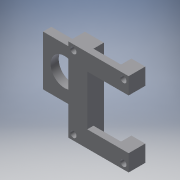
# Autodesk Inventor part: Bat_fixture
Saved by Autodesk Inventor 2019.3 (Build 233278000, 278)
## iProperties
Created: 2020-09-10
Part Number: Bat_fixture
Material: Generisch
Document SubType Name: Modeling
Designer: Nicolas Frick
Density: 1 g/cm^3
Appearance: Vorgabe
Author: Nicolas Frick
Autodesk Inventor part; units mm, degrees
ref_plane "YZ Plane" through (0, 0, 0) normal (1, 0, 0) x (0, 1, 0)
ref_plane "XZ Plane" through (0, 0, 0) normal (0, 1, 0) x (-1, 0, 0)
ref_plane "XY Plane" through (0, 0, 0) normal (0, 0, 1) x (1, 0, 0)
sketch "Skizze1" plane through (0, 0, 0) normal (0, 0, 1) x (1, 0, 0)
  line L0 (7.35, 100) -> (-7.35, 100) construction
  line L1 (-7.35, 0) -> (-7.35, 100) construction
  line L2 (7.35, 0) -> (-7.35, 0) construction
  line L3 (7.35, 0) -> (7.35, 100) construction
  circle A0 centre (-1.15, 77.5) radius 5.5 construction
  circle A1 centre (-1.15, 22.5) radius 5.5 construction
  circle A2 centre (-1.15, 93.5) radius 3.3 construction
  circle A3 centre (-1.15, 6.5) radius 3.3 construction
  line L4 (65.05, 100) -> (50.35, 100) construction
  line L5 (50.35, 0) -> (50.35, 100) construction
  line L6 (65.05, 0) -> (50.35, 0) construction
  line L7 (65.05, 0) -> (65.05, 100) construction
  circle A4 centre (58.85, 77.5) radius 5.5 construction
  circle A5 centre (58.85, 22.5) radius 5.5 construction
  circle A6 centre (58.85, 93.5) radius 3.3 construction
  circle A7 centre (58.85, 6.5) radius 3.3 construction
  line L8 (15.4049, 37.5868) -> (15.4049, 77.5868) construction
  line L9 (42.4049, 37.5868) -> (42.4049, 77.5868) construction
  line L10 (-7.35, 100) -> (65.05, 100)
  line L11 (65.05, 100) -> (65.05, 80)
  line L12 (65.05, 80) -> (-7.35, 80)
  line L13 (-7.35, 80) -> (-7.35, 100)
  line L14 (65.05, 0) -> (-7.35, 0)
  line L15 (-7.35, 0) -> (-7.35, 20)
  line L16 (-7.35, 20) -> (65.05, 20)
  line L17 (65.05, 20) -> (65.05, 0)
  circle A8 centre (-26.825, 50.9692) radius 16.4871 construction
  line L18 (15.4049, 80) -> (-52.5951, 80)
  line L19 (-52.5951, 80) -> (-52.5951, 20)
  line L20 (-52.5951, 20) -> (15.4049, 20)
  line L21 (15.4049, 20) -> (15.4049, 80)
  circle A9 centre (-26.825, 50.9692) radius 16.7
  point P0 (0, 0)
  point P1 (16.9249, 55.5859)
  dimension "d3" = 33.4
  constraints: 24 end point, 6 parallel, 4 point on line, 3 horizontal, 3 perpendicular, 1 centre point, 1 coincident, 1 other
  measures "d3" diameter of A9
extrude "Extrusion1" add sketch "Skizze1" along normal blind 20
sketch "Skizze2" plane through (0, 0, 20) normal (0, 0, 1) x (1, 0, 0)
  circle A0 centre (-1.15, 93.5) radius 2.5 projected
  circle A1 centre (58.85, 93.5) radius 2.5 projected
  circle A2 centre (-1.15, 6.5) radius 2.5 projected
  circle A3 centre (58.85, 6.5) radius 2.5 projected
  point P0 (0, 0)
hole "Bohrung1" at (-1.15, 93.5, 20) at (58.85, 93.5, 20) at (58.85, 6.5, 20) at (-1.15, 6.5, 20) direction (0, 0, -1) diameter 4.3 end through all counterbore diameter 7.3 counterbore depth 7.5
sketch "Skizze3" plane through (-7.35, 0, 0) normal (0, -1, 0) x (1, 0, 0)
  line L0 (46.2, -6) -> (72.4, -6) construction
  line L1 (72.7, -7.2) -> (72.7, -21.5) construction
  line L2 (46.7, -7.2) -> (46.7, -16.5) construction
  line L3 (25.7, -7.2) -> (25.7, -16.5) construction
  line L4 (-0.3, -7.2) -> (-0.3, -21.5) construction
  line L5 (116.8014, -58) -> (115.3014, -58) projected
  line L6 (72.4, 0) -> (57.7, 0) construction
  line L7 (14.7, 0) -> (0, 0) construction
  line L8 (72.4, 0) -> (0, 0) construction
  line L9 (2.55, 20) -> (9.85, 20) construction
  line L10 (62.55, 20) -> (69.85, 20) construction
  line L11 (49.7549, 2.5) -> (49.7549, 8.5) construction
  line L12 (48.2349, 2.5) -> (49.5076, 2.5) construction
  line L13 (72.4, 0) -> (0, 0) construction
  line L14 (72.4, 0) -> (72.4, 20) construction
  line L15 (0, 20) -> (72.4, 20) construction
  line L16 (0, 0) -> (0, 20) construction
  line L17 (22.7549, 8.6) -> (22.7549, 2.6) construction
  line L18 (23.1949, 8.9) -> (51.1949, 8.9) construction
  line L19 (51.1949, 1.6) -> (23.1949, 1.6) construction
  line L20 (55.7549, 12.5) -> (43.7549, 12.5)
  line L21 (0, 0) -> (72.4, 0) construction
  line L22 (43.7549, -12.5) -> (55.7549, 12.5) construction
  line L23 (55.7549, -12.5) -> (43.7549, 12.5) construction
  line L24 (43.7549, 0) -> (55.7549, 0)
  line L25 (55.7549, 0) -> (55.7549, 12.5)
  line L26 (22.7549, 0) -> (43.7549, 0)
  line L27 (43.7549, 12.5) -> (22.7549, 12.5)
  line L28 (22.7549, 12.5) -> (22.7549, 0)
  line L29 (22.7549, 12.5) -> (55.7549, 12.5)
  line L30 (55.7549, 12.5) -> (55.7549, 0)
  line L31 (55.7549, 0) -> (22.7549, 0)
  line L32 (22.7549, 0) -> (22.7549, 12.5)
  point P0 (7.35, 0)
  point P1 (49.7549, 0)
  constraints: 24 end point, 3 parallel, 2 horizontal, 2 midpoint, 1 perpendicular, 5 other
extrude "Extrusion2" cut sketch "Skizze3" against normal through all
sketch "Skizze4" plane through (0, 0, 20) normal (0, 0, 1) x (1, 0, 0)
  circle A0 centre (58.85, 6.5) radius 3.65 construction
  circle A1 centre (-1.15, 93.5) radius 3.65 construction
  circle A2 centre (58.85, 93.5) radius 3.65 construction
  circle A3 centre (-1.15, 6.5) radius 3.65 construction
  circle A4 centre (-26.825, 50.9692) radius 16.7 construction
  line L0 (65.05, 100) -> (-7.35, 100) construction
  line L1 (-7.35, 100) -> (-7.35, 80) construction
  line L2 (-7.35, 80) -> (-52.5951, 80) construction
  line L3 (-52.5951, 80) -> (-52.5951, 20) construction
  line L4 (-52.5951, 20) -> (-7.35, 20) construction
  line L5 (-7.35, 20) -> (-7.35, 0) construction
  line L6 (-7.35, 0) -> (65.05, 0) construction
  line L7 (65.05, 0) -> (65.05, 20) construction
  line L8 (65.05, 20) -> (15.4049, 20) construction
  line L9 (15.4049, 20) -> (15.4049, 80) construction
  line L10 (15.4049, 80) -> (65.05, 80) construction
  line L11 (65.05, 80) -> (65.05, 100) construction
  line L12 (-52.5951, 80) -> (-7.35, 80)
  line L13 (-7.35, 80) -> (-7.35, 20)
  line L14 (-7.35, 20) -> (-52.5951, 20)
  line L15 (-52.5951, 20) -> (-52.5951, 80)
  point P0 (0, 0)
  constraints: 8 end point, 2 parallel, 1 horizontal, 1 perpendicular
extrude "Extrusion3" cut sketch "Skizze4" against normal blind 15
sketch "Skizze5" plane through (0, 0, 0) normal (0, 0, -1) x (-1, 0, 0)
  line L0 (7.35, 20) -> (52.5951, 20) construction
  line L1 (52.5951, 20) -> (52.5951, 80) construction
  circle A0 centre (26.825, 50.9692) radius 30.5 construction
  line L2 (52.5951, 80) -> (7.35, 80) construction
  circle A1 centre (26.825, 50.9692) radius 17 projected
  line L3 (7.35, 80) -> (7.35, 20) projected
  line L4 (52.5951, 20) -> (7.35, 20)
  line L5 (7.35, 20) -> (7.35, 80)
  line L6 (7.35, 80) -> (52.5951, 80)
  line L7 (52.5951, 80) -> (52.5951, 20)
  point P0 (0, 0)
  constraints: 8 end point, 2 parallel, 1 horizontal, 1 perpendicular
extrude "Extrusion4" add sketch "Skizze5" along normal blind 5
